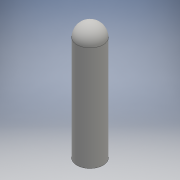
# Autodesk Inventor part: polaris_K05_screw
Saved by Autodesk Inventor 2016 (Build 200138000, 138)
## iProperties
Created: 2015-09-04
Part Number: polaris_K05_screw
Material: Generic
Document SubType Name: Modeling
Designer: HE BEC
Density: 1 g/cm^3
Appearance: Default
Author: HE BEC
Autodesk Inventor part; units mm, degrees
ref_plane "YZ Plane" through (0, 0, 0) normal (1, 0, 0) x (0, 1, 0)
ref_plane "XZ Plane" through (0, 0, 0) normal (0, 1, 0) x (-1, 0, 0)
ref_plane "XY Plane" through (0, 0, 0) normal (0, 0, 1) x (1, 0, 0)
sketch "Sketch1" plane through (0, 0, 0) normal (0, 0, 1) x (1, 0, 0)
  circle A0 centre (0, 0) radius 2
  dimension "d0" = 4
  constraints: 1 centre point, 1 coincident
  measures "d0" diameter of A0
extrude "Extrusion1" add sketch "Sketch1" along normal blind 16
sketch "Sketch3" plane through (0, 0, 16) normal (0, 0, 1) x (1, 0, 0)
  arc A0 (0, -2) -> (0, 2) centre (0, 0) ccw
  line L0 (0, 2) -> (0, -2)
  dimension "d4" = 4
  constraints: 2 end point, 2 point on circle, 1 centre point, 1 vertical
  measures "d4" diameter of A0
revolve "Revolution1" add sketch "Sketch3" angle 360 about axis through (0, 2, 16) along (0, -1, 0)
body "Solid1"
